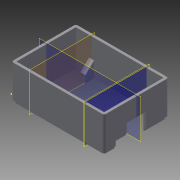
# Autodesk Inventor part: hubLid1.2
Saved by Autodesk Inventor 2015 (Build 190159000, 159)
## iProperties
Created: 2015-11-06
Part Number: hubLid1.2
Material: Generic
Document SubType Name: Modeling
Designer: mca20
Density: 1 g/cm^3
Appearance: Default
Author: mca20
Autodesk Inventor part; units mm, degrees
ref_plane "YZ Plane" through (0, 0, 0) normal (1, 0, 0) x (0, 1, 0)
ref_plane "XZ Plane" through (0, 0, 0) normal (0, 1, 0) x (-1, 0, 0)
ref_plane "XY Plane" through (0, 0, 0) normal (0, 0, 1) x (1, 0, 0)
sketch "Sketch2" plane through (0, 0, 0) normal (0, 1, 0) x (-1, 0, 0)
  line L0 (0, 0) -> (-92, 0)
  line L1 (-92, 0) -> (-92, -64)
  line L2 (-92, -64) -> (0, -64)
  line L3 (0, -64) -> (0, 0)
  line L4 (-89.5, -61.5) -> (-2.5, -61.5)
  line L5 (-2.5, -61.5) -> (-2.5, -2.5)
  line L6 (-2.5, -2.5) -> (-89.5, -2.5)
  line L7 (-89.5, -2.5) -> (-89.5, -61.5)
  dimension "d2" = 92
  dimension "d3" = 64
  dimension "d4" = 2.5
  dimension "d5" = 2.5
  dimension "d6" = 2.5
  dimension "d7" = 2.5
  constraints: 16 end point, 5 parallel, 2 horizontal, 2 perpendicular
  measures "d2" distance of L2.end L1.end
  measures "d3" distance of L1.end L0.end
  measures "d4" distance between parallel lines of L4 L2
  measures "d5" distance between parallel lines of L0 L6
  measures "d6" distance between parallel lines of L1 L7
  measures "d7" distance between parallel lines of L3 L5
extrude "Extrusion1" add sketch "Sketch2" along normal blind 32.5
sketch "Sketch3" plane through (0, 32.5, 0) normal (0, 1, 0) x (1, 0, 0)
  line L0 (0, 64) -> (0, 0) projected
  line L1 (92, 64) -> (0, 64) projected
  line L2 (92, 0) -> (92, 64) projected
  line L3 (0, 0) -> (92, 0) projected
extrude "Extrusion2" [suppressed]
fillet "Fillet1" radius 2 4 edges at (0, 16.25, 0) (92, 16.25, 0) (92, 16.25, -64) (0, 16.25, -64)
sketch "Sketch4" plane through (0, 0, 0) normal (0, -1, 0) x (1, 0, 0)
  line L0 (90.7, -1.3) -> (1.3, -1.3)
  line L1 (1.3, -1.3) -> (1.3, -62.7)
  line L2 (1.3, -62.7) -> (90.7, -62.7)
  line L3 (90.7, -62.7) -> (90.7, -1.3)
  line L4 (89.5, -2.5) -> (89.5, -61.5) projected
  line L5 (89.5, -61.5) -> (2.5, -61.5) projected
  line L6 (2.5, -61.5) -> (2.5, -2.5) projected
  line L7 (2.5, -2.5) -> (89.5, -2.5) projected
  point P0 (0, 0)
  constraints: 8 end point, 2 parallel, 1 horizontal, 1 perpendicular
extrude "Extrusion4" add sketch "Sketch4" along normal blind 2.5
sketch "Sketch6" plane through (0, -2.5, 0) normal (0, -1, 0) x (1, 0, 0)
  line L0 (73, -8.5) -> (18, -8.5)
  line L1 (18, -8.5) -> (18, -55.5)
  line L2 (18, -55.5) -> (73, -55.5)
  line L3 (73, -55.5) -> (73, -8.5)
  line L4 (88, -2.5) -> (0.5, -2.5)
  line L5 (88, -61.5) -> (0.5, -61.5)
  line L6 (88, -2.5) -> (88, -61.5)
  line L7 (0.5, -61.5) -> (0.5, -2.5)
  line L8 (75.5, -2.5) -> (70.5, -2.5)
  line L9 (70.5, -2.5) -> (70.5, -11)
  line L10 (70.5, -11) -> (75.5, -11)
  line L11 (75.5, -11) -> (75.5, -2.5)
  line L12 (74.5, -61.5) -> (69.5, -61.5)
  line L13 (69.5, -61.5) -> (69.5, -53)
  line L14 (69.5, -53) -> (74.5, -53)
  line L15 (74.5, -53) -> (74.5, -61.5)
  line L16 (20.5, -2.5) -> (15.5, -2.5)
  line L17 (15.5, -2.5) -> (15.5, -11)
  line L18 (15.5, -11) -> (20.5, -11)
  line L19 (20.5, -11) -> (20.5, -2.5)
  line L20 (20.5, -53) -> (15.5, -53)
  line L21 (15.5, -53) -> (15.5, -61.5)
  line L22 (15.5, -61.5) -> (20.5, -61.5)
  line L23 (20.5, -61.5) -> (20.5, -53)
  line L24 (72, -8.5) -> (72, -55.5)
  line L25 (89.5, -2.5) -> (89.5, -61.5) projected
  line L26 (2.5, -61.5) -> (2.5, -2.5) projected
  point P0 (0, 0)
  dimension "d17" = 6
  dimension "d18" = 6
  dimension "d22" = 5
  dimension "d23" = 8.5
  dimension "d24" = 0
  dimension "d25" = 5
  dimension "d26" = 8.5
  dimension "d27" = 0
  dimension "d28" = 5
  dimension "d29" = 8.5
  dimension "d30" = 0
  dimension "d31" = 2.5
  dimension "d34" = 5
  dimension "d35" = 8.5
  dimension "d36" = 0
  dimension "d37" = 2.5
  dimension "d38" = 2.5
  dimension "d39" = 1
  dimension "d40" = 2.5
  dimension "d86" = 16.5
  dimension "d89" = 15.5
  dimension "d109" = 17.5
  constraints: 50 end point, 10 parallel, 6 perpendicular, 5 horizontal, 2 point on line
  measures "d17" distance between parallel lines of L4 L0
  measures "d18" distance between parallel lines of L5 L2
  measures "d22" distance of L10.end L9.end
  measures "d23" distance of L9.end L8.end
  measures "d24" distance between parallel lines of L4 L8
  measures "d25" distance of L13.end L14.end
  measures "d26" distance of L12.end L13.end
  measures "d27" distance between parallel lines of L5 L12
  measures "d28" distance of L18.end L17.end
  measures "d29" distance of L17.end L16.end
  measures "d30" distance between parallel lines of L4 L16
  measures "d31" distance between parallel lines of L9 L3
  measures "d34" distance of L22.end L21.end
  measures "d35" distance of L21.end L20.end
  measures "d36" distance between parallel lines of L5 L22
  measures "d37" distance from line of L1 L20.start
  measures "d38" distance between parallel lines of L19 L1
  measures "d39" distance between parallel lines of L24 L3
  measures "d40" distance between parallel lines of L15 L24
  measures "d86" distance from line of L25 L0.start
  measures "d89" distance between parallel lines of L26 L1
  measures "d109" distance between parallel lines of L25 L24
extrude "Extrusion5" add sketch "Sketch6" against normal blind 7 contours L3 L10 L24 L0 | L0 L9 L4 L11 L10 L3 | L24 L10 L9 L0 | L14 L15 L5 L13 L2 L3 | L3 L2 L24 L14 | L19 L18 L1 L0 | L0 L1 L18 L17 L4 L19 | L24 L2 L13 L14 | L20 L23 L2 L1 | L1 L2 L23 L5 L21 L20
sketch "Sketch8" plane through (0, -2.5, 0) normal (0, -1, 0) x (1, 0, 0)
  circle A0 centre (73, -8) radius 1.5
  line L0 (70.5, -2.5) -> (70.5, -11) projected
  circle A1 centre (18, -8) radius 1.5
  line L1 (15.5, -2.5) -> (15.5, -11) projected
  circle A2 centre (18, -56) radius 1.5
  circle A3 centre (72, -56) radius 1.5
  line L2 (2, 0) -> (90, 0) projected
  line L3 (69.5, -61.5) -> (69.5, -53) projected
  line L4 (90, -64) -> (2, -64) projected
  line L5 (15.5, -53) -> (15.5, -61.5) projected
  line L6 (89.5, -61.5) -> (89.5, -2.5) projected
  line L7 (2.5, -61.5) -> (2.5, -2.5) projected
  point P0 (0, 0)
  dimension "d47" = 3
  dimension "d48" = 2.5
  dimension "d49" = 3
  dimension "d50" = 2.5
  dimension "d51" = 3
  dimension "d52" = 3
  dimension "d53" = 8
  dimension "d54" = 2.5
  dimension "d55" = 8
  dimension "d56" = 8
  dimension "d57" = 2.5
  dimension "d58" = 8
  dimension "d108" = 15.5
  constraints: 4 centre point
  measures "d47" diameter of A0
  measures "d48" distance from line of L0 A0.centre
  measures "d49" diameter of A1
  measures "d50" distance from line of L1 A1.centre
  measures "d51" diameter of A2
  measures "d52" diameter of A3
  measures "d53" distance from line of L2 A0.centre
  measures "d54" distance from line of A3.centre L3
  measures "d55" distance from line of L2 A1.centre
  measures "d56" distance from line of L4 A3.centre
  measures "d57" distance from line of L5 A2.centre
  measures "d58" distance from line of L4 A2.centre
  measures "d108" distance from line of L7 A2.centre
hole "Hole1" at (73, -2.5, -8) at (72, -2.5, -56) at (18, -2.5, -56) at (18, -2.5, -8) direction (0, 1, 0) diameter 3 depth 5
sketch "Sketch9" plane through (92, 0, -2) normal (1, 0, 0) x (0, 0, -1)
  line L0 (60.7, -2.5) -> (-0.7, -2.5) projected
  line L1 (9.5, 14.5) -> (39.5, 14.5)
  line L2 (39.5, 14.5) -> (39.5, -2.5)
  line L3 (39.5, -2.5) -> (9.5, -2.5)
  line L4 (9.5, -2.5) -> (9.5, 14.5)
  line L5 (59.5, 32.5) -> (59.5, -2.5) projected
  line L6 (0.5, -2.5) -> (0.5, 32.5) projected
  line L7 (9.5, 14.5) -> (20.5, 14.5)
  line L8 (20.5, 14.5) -> (20.5, 4.5)
  line L9 (20.5, 4.5) -> (9.5, 4.5)
  line L10 (9.5, 4.5) -> (9.5, 14.5)
  point P0 (-2, 0)
  dimension "d66" = 20
  dimension "d67" = 9
  dimension "d68" = 17
  dimension "d69" = 11
  dimension "d70" = 10
  constraints: 16 end point, 4 parallel, 2 horizontal, 2 perpendicular, 1 point on line
  measures "d66" distance between parallel lines of L5 L2
  measures "d67" distance between parallel lines of L6 L4
  measures "d68" distance between parallel lines of L0 L1
  measures "d69" distance of L8.end L9.end
  measures "d70" distance of L7.end L8.end
extrude "Extrusion6" cut sketch "Sketch9" against normal blind 5 contours L0 L4 L9 L8 L1 L2
fillet "Fillet2" radius 2 1 edges at (90.75, 4.5, -22.5)
sketch "Sketch10" plane through (0, 4.5, 0) normal (0, 1, 0) x (1, 0, 0)
  point P0 (0, 0)
ref_plane "Work Plane1" through (18, 32.5, -2.5) normal (1, 0, 0) x (0, 0, -1)
sketch "Sketch12" plane through (18, 32.5, -2.5) normal (1, 0, 0) x (0, 0, -1)
  line L0 (50.5, -28) -> (59.4936, -19.0064)
  line L1 (50.5, -28) -> (63.2188, -28) construction
  point P0 (-2.5, -32.5)
  dimension "d98" = 45
  constraints: 4 end point, 1 equal length, 1 horizontal
  measures "d98" angle of L1 L0
extrude "Rib1" add sketch "Sketch12" along normal mid plane 5 rib yes fills toward (55.0321, -23.5386) open curves L0
ref_plane "Work Plane2" through (89.5, 32.5, -32) normal (0, 0, -1) x (-1, 0, 0)
mirror "Mirror1" about plane through (89.5, 32.5, -32) normal (0, 0, -1) of "Rib1"
ref_plane "Work Plane4" through (72, 32.5, -61.5) normal (-1, 0, 0) x (0, 0, 1)
sketch "Sketch14" plane through (72, 32.5, -61.5) normal (-1, 0, 0) x (0, 0, 1)
  line L0 (8.5, -28) -> (4, -23.5)
  line L1 (8.5, -28) -> (14.864, -28) construction
  point P0 (61.5, -32.5)
  dimension "d97" = 135
  constraints: 4 end point, 1 equal length, 1 horizontal
  measures "d97" angle of L1 L0
extrude "Rib2" add sketch "Sketch14" along normal mid plane 5 rib yes fills toward (6.2146, -25.7854) open curves L0
ref_plane "Work Plane5" through (73, 32.5, -61.5) normal (-1, 0, 0) x (0, 0, 1)
sketch "Sketch15" plane through (73, 32.5, -61.5) normal (-1, 0, 0) x (0, 0, 1)
  line L0 (50.5, -28.3198) -> (57.3483, -28.3198) construction
  line L1 (50.5, -28) -> (55.1214, -23.3786)
  line L2 (50.5, -28) -> (57.0356, -28) construction
  point P0 (61.5, -32.5)
  dimension "d101" = 45
  constraints: 6 end point, 2 horizontal, 1 equal length
  measures "d101" angle of L2 L1
extrude "Rib3" add sketch "Sketch15" along normal mid plane 5 rib yes fills toward (52.846, -25.7247) open curves L1
fillet "Fillet3" radius 2 4 edges at (90.7, -1.25, -1.3) (90.7, -1.25, -62.7) (1.3, -1.25, -62.7) (1.3, -1.25, -1.3)
equation "\"d5\" = d4"
equation "\"d6\" = d4"
equation "\"d7\" = d4"
equation "\"d18\" = d17"
equation "\"d37\" = d33"
equation "\"d38\" = d37"
equation "\"d40\" = d31"
equation "\"d49\" = d47"
equation "\"d50\" = d48"
equation "\"d51\" = d47"
equation "\"d52\" = d47"
equation "\"d54\" = d48"
equation "\"d55\" = d53"
equation "\"d56\" = d53"
equation "\"d57\" = d48"
equation "\"d58\" = d53"
equation "\"d33\" = d31"
body "Solid1"
